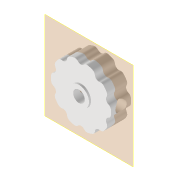
# Autodesk Inventor part: 00_Turningscrew
Saved by Autodesk Inventor 2022 (Build 260153000, 153)
## iProperties
Created: 2023-05-12
Part Number: 00_Turningscrew
Material: Generisch
Document SubType Name: Modeling
Designer: diederichbenedict
Density: 1 g/cm^3
Appearance: Vorgabe
Author: diederichbenedict
Autodesk Inventor part; units mm, degrees
ref_plane "YZ Plane" through (0, 0, 0) normal (1, 0, 0) x (0, 1, 0)
ref_plane "XZ Plane" through (0, 0, 0) normal (0, 1, 0) x (-1, 0, 0)
ref_plane "XY Plane" through (0, 0, 0) normal (0, 0, 1) x (1, 0, 0)
sketch "Skizze1" plane through (0, 0, 0) normal (0, 0, 1) x (1, 0, 0)
  circle A0 centre (0, 0) radius 1.45
  circle A1 centre (0, 0) radius 7.5
  dimension "d0" = 2.9
  dimension "d1" = 15
  constraints: 2 centre point, 2 coincident
  measures "d0" diameter of A0
  measures "d1" diameter of A1
extrude "Extrusion1" add sketch "Skizze1" along normal blind 5
ref_plane "Arbeitsebene1" through (0, 0, 3) normal (0, 0, 1) x (1, 0, 0)
sketch "Skizze2" plane through (0, 0, 5) normal (0, 0, 1) x (1, 0, 0)
  circle A0 centre (0, 0) radius 7.5 projected
  circle A1 centre (0, 0) radius 7.5 projected
  line L0 (0, 0) -> (0, 7.5)
  line L1 (0, 5.8923) -> (1.0718, 7.423)
  line L2 (0, 5.8923) -> (1.8686, 5.8923) construction
  line L3 (1.0718, 7.423) -> (0, 5.8923)
  line L4 (0, 5.8923) -> (-1.0718, 7.423)
  line L5 (0, 5.8923) -> (1.8686, 5.8923) construction
  dimension "d17" = 55
  dimension "d18" = 125
  constraints: 12 end point, 3 point on circle, 2 equal length, 2 horizontal, 1 collinear, 1 point on line, 1 vertical
  measures "d17" angle of L2 L1
  measures "d18" angle of L5 L4
extrude "Extrusion2" cut sketch "Skizze2" against normal blind 5 contours L1 L0 A0 | A0 L0 L4
sketch "Skizze5" plane through (0, 0, 5) normal (0, 0, 1) x (1, 0, 0)
  circle A0 centre (0, 0) radius 1.45 projected
  circle A1 centre (0, 0) radius 2.5
  dimension "d14" = 5
  constraints: 1 centre point, 1 coincident
  measures "d14" diameter of A1
extrude "Extrusion4" add sketch "Skizze5" along normal blind 0.5
fillet "Rundung2" radius 1 3 edges at (1.0718, 7.423, 2.5) (-1.0718, 7.423, 2.5) (0, 5.8923, 2.5)
pattern_circular "Runde Anordnung3" count 10 over 360 about axis through (0, 0, 0) along (0, 0, 1) of "Rundung2", "Extrusion2"
sketch "Skizze6" plane through (0, 0, 0) normal (1, 0, 0) x (0, 1, 0)
  line L0 (-1.5, -2.9) -> (-1.5, 21.6933)
  line L1 (1.5, -2.9) -> (1.5, 21.6933)
  line L2 (-1.5, 0) -> (1.5, 0)
  line L3 (-1.5, 1) -> (1.5, 1)
  circle A0 centre (0, 2.5) radius 1.5
  circle A1 centre (0, 2.5) radius 1.4
  point P0 (0, 0)
  dimension "d26" = 2.5
  dimension "d27" = 2.8
  constraints: 8 end point, 4 point on line, 3 tangent, 2 centre point, 2 perpendicular, 2 vertical, 1 coincident, 4 other
  measures "d26" distance of A0.centre point (0, 0)
  measures "d27" diameter of A1
extrude "Extrusion5" cut sketch "Skizze6" along normal through all both and the other way through all contours A1
